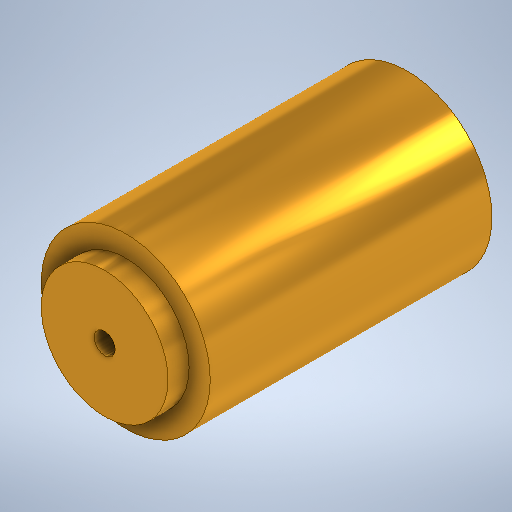
# Autodesk Inventor part: 153 part 1
Saved by Autodesk Inventor 2025.1 (Build 291241000, 241)
## iProperties
Created: 2024-08-01
Part Number: 153 part 1
Material: Gold
Document SubType Name: Modeling
Designer: ffogue
Density: 19.3 g/cm^3
Appearance: Metal 1800F Hot
Author: ffogue
Autodesk Inventor part; units mm, degrees
ref_plane "YZ Plane" through (0, 0, 0) normal (1, 0, 0) x (0, 1, 0)
ref_plane "XZ Plane" through (0, 0, 0) normal (0, 1, 0) x (-1, 0, 0)
ref_plane "XY Plane" through (0, 0, 0) normal (0, 0, 1) x (1, 0, 0)
sketch "Skizze2" plane through (0, 0, 0) normal (0, 0, 1) x (1, 0, 0)
  line L0 (0, 0) -> (4.5, 0)
  line L1 (4.5, 0) -> (4.5, 1.5)
  line L2 (4.5, 1.5) -> (6, 1.5)
  line L3 (6, 1.5) -> (6, 21.5)
  line L4 (6, 21.5) -> (0, 21.5)
  line L5 (0, 21.5) -> (0, 0)
  point P0 (2.25, 0)
  point P1 (5.25, 1.5)
  dimension "d1" = 21.5
  dimension "d2" = 1.5
  dimension "d3" = 12
  dimension "d4" = 9
  constraints: 12 end point, 5 perpendicular, 2 midpoint, 1 horizontal
  measures "d1" distance from line of point (2.25, 0) L4
  measures "d2" distance from line of L0 point (5.25, 1.5)
  measures "d3" diameter of L3 L5
  measures "d4" diameter of L1 L5
revolve "Umdrehung1" add sketch "Skizze2" angle 360 about axis through (0, 21.5, 0) along (0, -1, 0)
sketch "Skizze3" plane through (0, 21.5, 0) normal (0, 1, 0) x (1, 0, 0)
  circle A0 centre (0, 0) radius 6 projected
  constraints: 1 coincident
hole "Bohrung1" at (0, 21.5, 0) direction (0, -1, 0) diameter 8 depth 18
sketch "Sketch4" plane through (0, 0, 0) normal (0, -1, 0) x (1, 0, 0)
  circle A0 centre (0, 0) radius 4.5 projected
  constraints: 1 coincident
hole "Hole2" at (0, 0, 0) direction (0, 1, 0) diameter 1.5 depth 1.5
